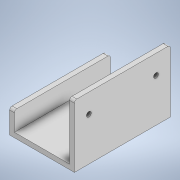
# Autodesk Inventor part: Ozone Holder
Saved by Autodesk Inventor 2021 (Build 250183000, 183)
## iProperties
Created: 2020-09-05
Part Number: Ozone Holder
Material: Generic
Document SubType Name: Modeling
Designer: cmzgt
Density: 1 g/cm^3
Appearance: Default
Author: cmzgt
## iProperties of the stored document _3DPrint.ipt
Created: 2020-09-05
Part Number: _3DPrint
Material: Generic
Document SubType Name: Modeling
Designer: cmzgt
Density: 1 g/cm^3
Appearance: Default
Author: cmzgt
Autodesk Inventor part; units mm, degrees
note: some values were not read from the file. Chosen so that the rebuilt part matches the saved one: direction of "Emboss1".
ref_plane "YZ Plane" through (0, 0, 0) normal (1, 0, 0) x (0, 1, 0)
ref_plane "XZ Plane" through (0, 0, 0) normal (0, 1, 0) x (-1, 0, 0)
ref_plane "XY Plane" through (0, 0, 0) normal (0, 0, 1) x (1, 0, 0)
sketch "Sketch1" plane through (0, 0, 0) normal (0, 1, 0) x (-1, 0, 0)
  line L0 (-42.8625, -63.5) -> (42.8625, -63.5)
  line L1 (42.8625, -63.5) -> (42.8625, 63.5)
  line L2 (42.8625, 63.5) -> (-42.8625, 63.5)
  line L3 (-42.8625, 63.5) -> (-42.8625, -63.5)
  line L4 (-42.8625, -63.5) -> (42.8625, 63.5) construction
  line L5 (42.8625, -63.5) -> (-42.8625, 63.5) construction
  point P0 (0, 0)
  dimension "d0" = 85.725
  dimension "d1" = 127
  constraints: 12 end point, 2 midpoint, 2 parallel, 1 horizontal, 1 perpendicular
  measures "d0" distance of L2.end L1.end
  measures "d1" distance of L0.end L1.end
extrude "Extrusion1" add sketch "Sketch1" along normal blind 6.35
sketch "Sketch2" plane through (0, 6.35, 0) normal (0, 1, 0) x (1, 0, 0)
  line L0 (-42.8625, 63.5) -> (-42.8625, -63.5) projected
  line L1 (42.8625, 63.5) -> (-42.8625, 63.5) projected
  line L2 (-42.8625, -63.5) -> (-36.5125, -63.5)
  line L3 (-36.5125, -63.5) -> (-36.5125, 63.5)
  line L4 (-36.5125, 63.5) -> (-42.8625, 63.5)
  line L5 (-42.8625, 63.5) -> (-42.8625, -63.5)
  point P0 (0, 0)
  dimension "d4" = 6.35
  constraints: 8 end point, 2 parallel, 1 horizontal, 1 perpendicular, 1 point on line
  measures "d4" distance of L4.end L3.end
extrude "Extrusion2" add sketch "Sketch2" along normal blind 25.4
sketch "Sketch3" plane through (0, 6.35, 0) normal (0, 1, 0) x (1, 0, 0)
  line L0 (42.8625, -63.5) -> (42.8625, 63.5) projected
  line L1 (42.8625, 63.5) -> (-42.8625, 63.5) projected
  line L2 (42.8625, -63.5) -> (36.5125, -63.5)
  line L3 (36.5125, -63.5) -> (36.5125, 63.5)
  line L4 (36.5125, 63.5) -> (42.8625, 63.5)
  line L5 (42.8625, 63.5) -> (42.8625, -63.5)
  point P0 (0, 0)
  dimension "d7" = 6.35
  constraints: 8 end point, 2 parallel, 1 horizontal, 1 perpendicular, 1 point on line
  measures "d7" distance of L3.end L4.end
extrude "Extrusion3" add sketch "Sketch3" along normal blind 76.2
sketch "Sketch4" plane through (42.8625, 0, 63.5) normal (1, 0, 0) x (0, 0, -1)
  circle A0 centre (19.05, 57.15) radius 3.175
  line L0 (0, 82.55) -> (127, 82.55) projected
  line L1 (0, 0) -> (0, 82.55) projected
  line L2 (127, 82.55) -> (0, 82.55) construction
  line L3 (63.5, 82.55) -> (63.5, 0) construction
  line L4 (127, 0) -> (0, 0) construction
  circle A1 centre (107.95, 57.15) radius 3.175
  dimension "d10" = 6.35
  dimension "d11" = 25.4
  dimension "d12" = 19.05
  constraints: 2 centre point, 2 end point, 1 midpoint, 1 perpendicular, 1 symmetric about line, 1 other
  measures "d10" diameter of A0
  measures "d11" distance from line of L0 A0.centre
  measures "d12" distance from line of L1 A0.centre
extrude "Extrusion4" cut sketch "Sketch4" against normal blind 76.2
fillet "Fillet1" radius 3.175 2 edges at (-39.6875, 31.75, -63.5) (-39.6875, 31.75, 63.5)
sketch "Sketch5" plane through (-42.8625, 0, -63.5) normal (-1, 0, 0) x (0, 0, 1)
  line L0 (26.6686, 23.4082) -> (100.3286, 23.4082) construction
  line L1 (100.3286, 23.4082) -> (100.3286, 10.7402) construction
  line L2 (100.3286, 10.7402) -> (26.6686, 10.7402) construction
  line L3 (26.6686, 10.7402) -> (26.6686, 23.4082) construction
  line L4 (63.5, 0) -> (63.5, 31.75) construction
  line L5 (3.175, 31.75) -> (123.825, 31.75) construction
  line L6 (0, 0) -> (0, 28.575) construction
  line L7 (38.8687, 23.4082) -> (42.9757, 23.4082)
  line L8 (42.9757, 23.4082) -> (45.8482, 14.2652)
  line L9 (45.8482, 14.2652) -> (48.6595, 23.4082)
  line L10 (48.6595, 23.4082) -> (52.6443, 23.4082)
  line L11 (52.6443, 23.4082) -> (47.9261, 10.7082)
  line L12 (47.9261, 10.7082) -> (43.6724, 10.7082)
  line L13 (43.6724, 10.7082) -> (38.8687, 23.4082)
  line L14 (53.8422, 19.9123) -> (57.3747, 19.9123)
  line L15 (57.3747, 19.9123) -> (57.3747, 10.7082)
  line L16 (57.3747, 10.7082) -> (53.8422, 10.7082)
  line L17 (53.8422, 10.7082) -> (53.8422, 19.9123)
  line L18 (53.8422, 23.4082) -> (57.3747, 23.4082)
  line L19 (57.3747, 23.4082) -> (57.3747, 21.0124)
  line L20 (57.3747, 21.0124) -> (53.8422, 21.0124)
  line L21 (53.8422, 21.0124) -> (53.8422, 23.4082)
  line L22 (66.4933, 14.3141) -> (69.8425, 13.9351)
  spline S0 degree 2 poles (69.8425, 13.9351) (69.5613, 12.8839) (68.3023, 11.356) (66.3344, 10.5004) (64.8187, 10.5004) knots 0 0 0 1 2 3 3 3
  spline S1 degree 2 poles (64.8187, 10.5004) (63.3519, 10.5004) (61.3962, 11.0504) (59.9905, 12.2728) (59.196, 13.9107) (59.196, 15.2675) knots 0 0 0 1 2 3 4 4 4
  spline S2 degree 2 poles (59.196, 15.2675) (59.196, 16.6854) (59.6849, 17.6388) knots 0 0 0 1 1 1
  spline S3 degree 2 poles (59.6849, 17.6388) (60.0394, 18.3233) (61.274, 19.4234) (61.9218, 19.6923) knots 0 0 0 1 2 2 2
  spline S4 degree 2 poles (61.9218, 19.6923) (62.9485, 20.1201) (64.562, 20.1201) knots 0 0 0 1 1 1
  spline S5 degree 2 poles (64.562, 20.1201) (66.8111, 20.1201) (69.1824, 18.5066) (69.6591, 16.9543) knots 0 0 0 1 2 2 2
  line L23 (69.6591, 16.9543) -> (66.3344, 16.5143)
  spline S6 degree 2 poles (66.3344, 16.5143) (66.1755, 17.101) (65.3565, 17.6999) (64.6598, 17.6999) knots 0 0 0 1 2 2 2
  spline S7 degree 2 poles (64.6598, 17.6999) (63.792, 17.6999) (62.7041, 16.4531) (62.7041, 15.1819) knots 0 0 0 1 2 2 2
  spline S8 degree 2 poles (62.7041, 15.1819) (62.7041, 14.0451) (63.7797, 12.8717) (64.6109, 12.8717) knots 0 0 0 1 2 2 2
  spline S9 degree 2 poles (64.6109, 12.8717) (65.3076, 12.8717) (66.2611, 13.5807) (66.4933, 14.3141) knots 0 0 0 1 2 2 2
  line L24 (71.4682, 23.4082) -> (75.0741, 23.4082)
  line L25 (75.0741, 23.4082) -> (75.0741, 16.8687)
  line L26 (75.0741, 16.8687) -> (77.7021, 19.9123)
  line L27 (77.7021, 19.9123) -> (82.0413, 19.9123)
  line L28 (82.0413, 19.9123) -> (78.741, 16.6854)
  line L29 (78.741, 16.6854) -> (82.2369, 10.7082)
  line L30 (82.2369, 10.7082) -> (78.2643, 10.7082)
  line L31 (78.2643, 10.7082) -> (76.3942, 14.3874)
  line L32 (76.3942, 14.3874) -> (75.0741, 13.104)
  line L33 (75.0741, 13.104) -> (75.0741, 10.7082)
  line L34 (75.0741, 10.7082) -> (71.4682, 10.7082)
  line L35 (71.4682, 10.7082) -> (71.4682, 23.4082)
  line L36 (83.447, 19.9123) -> (86.9795, 19.9123)
  line L37 (86.9795, 19.9123) -> (86.9795, 10.7082)
  line L38 (86.9795, 10.7082) -> (83.447, 10.7082)
  line L39 (83.447, 10.7082) -> (83.447, 19.9123)
  line L40 (83.447, 23.4082) -> (86.9795, 23.4082)
  line L41 (86.9795, 23.4082) -> (86.9795, 21.0124)
  line L42 (86.9795, 21.0124) -> (83.447, 21.0124)
  line L43 (83.447, 21.0124) -> (83.447, 23.4082)
  dimension "d16" = 73.66
  dimension "d17" = 26.6686
  constraints: 2 end point, 1 midpoint, 2 other
  measures "d16" distance of L0.start L0.end
  measures "d17" distance between parallel lines of L6 L3
emboss "Emboss1" sketch "Sketch5" operation cut depth 1.5875 direction (1, 0, 0)
fillet "Fillet2" radius 3.175 2 edges at (39.6875, 82.55, -63.5) (39.6875, 82.55, 63.5)
body "Solid1"
